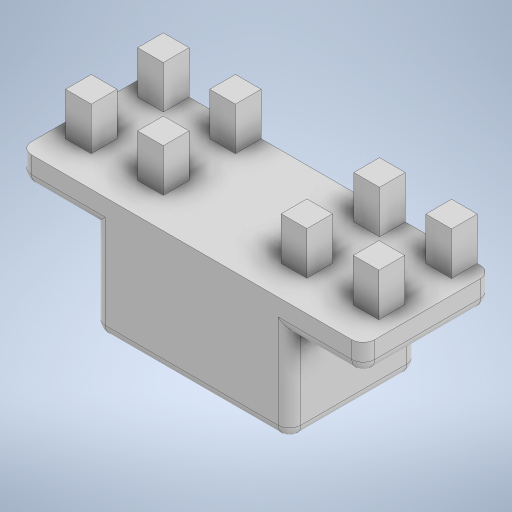
# Autodesk Inventor part: Platform
Saved by Autodesk Inventor 2024.1 (Build 281209000, 209)
## iProperties
Created: 2024-04-30
Part Number: Platform
Material: Generic
Document SubType Name: Modeling
Designer: cyan924
Density: 1 g/cm^3
Appearance: Default
Author: cyan924
Autodesk Inventor part; units mm, degrees
ref_plane "YZ Plane" through (0, 0, 0) normal (1, 0, 0) x (0, 1, 0)
ref_plane "XZ Plane" through (0, 0, 0) normal (0, 1, 0) x (-1, 0, 0)
ref_plane "XY Plane" through (0, 0, 0) normal (0, 0, 1) x (1, 0, 0)
sketch "Sketch1" plane through (0, 0, 0) normal (0, 1, 0) x (-1, 0, 0)
  line L0 (0, 0) -> (34.2, 0)
  line L1 (34.2, 0) -> (34.2, -22.5)
  line L2 (34.2, -22.5) -> (0, -22.5)
  line L3 (0, -22.5) -> (0, 0)
  line L4 (5, -17.5) -> (29.2, -17.5)
  line L5 (29.2, -17.5) -> (29.2, -5)
  line L6 (29.2, -5) -> (5, -5)
  line L7 (5, -5) -> (5, -17.5)
  dimension "d64" = 24.2
  dimension "d65" = 12.5
  dimension "d66" = 5
  dimension "d67" = 5
  dimension "d68" = 5
  dimension "d69" = 5
  constraints: 16 end point, 4 parallel, 2 horizontal, 2 perpendicular
  measures "d64" distance between parallel lines of L5 L7
  measures "d65" distance of L4.end L5.end
  measures "d66" distance between parallel lines of L1 L5
  measures "d67" distance between parallel lines of L3 L7
  measures "d68" distance between parallel lines of L0 L6
  measures "d69" distance between parallel lines of L2 L4
extrude "Extrusion4" add sketch "Sketch1" along normal blind 16.4
sketch "Sketch6" plane through (0, 16.4, 0) normal (0, 1, 0) x (1, 0, 0)
  line L0 (0, 0) -> (0, 22.5) projected
  line L1 (-34.2, 0) -> (0, 0) projected
  line L2 (-47.1, 22.5) -> (12.9, 22.5)
  line L3 (12.9, 22.5) -> (12.9, 0)
  line L4 (12.9, 0) -> (-47.1, 0)
  line L5 (-47.1, 0) -> (-47.1, 22.5)
  line L6 (0, 22.5) -> (-34.2, 22.5) projected
  point P0 (-17.1, 0)
  point P1 (15.9799, 21.8)
  point P2 (-17.1, 22.5)
  point P3 (-17.1, 22.5)
  dimension "d75" = 60
  dimension "d77" = 0
  constraints: 8 end point, 2 midpoint, 2 parallel, 1 horizontal, 1 perpendicular, 2 other
  measures "d75" distance between parallel lines of L3 L5
  measures "d77" distance of point (-17.1, 22.5) point (-17.1, 22.5)
extrude "Extrusion6" add sketch "Sketch6" along normal blind 5
sketch "Sketch7" plane through (0, 21.4, 0) normal (0, 1, 0) x (1, 0, 0)
  line L0 (-47.1, 22.5) -> (-47.1, 0) projected
  line L1 (-6.75, 22.5) -> (-6.75, 18)
  line L2 (-2.25, 22.5) -> (-2.25, 18)
  line L3 (-2.25, 18) -> (-6.75, 18)
  line L4 (-6.75, 22.5) -> (-2.25, 22.5)
  line L5 (12.9, 22.5) -> (-47.1, 22.5) projected
  line L6 (-31.95, 22.5) -> (-31.95, 18)
  line L7 (-27.45, 22.5) -> (-27.45, 18)
  line L8 (-27.45, 18) -> (-31.95, 18)
  line L9 (-31.95, 22.5) -> (-27.45, 22.5)
  line L10 (-40.05, 22.5) -> (-40.05, 18)
  line L11 (-40.05, 18) -> (-44.55, 18)
  line L12 (-44.55, 22.5) -> (-44.55, 18)
  line L13 (-44.55, 22.5) -> (-40.05, 22.5)
  line L14 (10.35, 22.5) -> (10.35, 18)
  line L15 (5.85, 22.5) -> (5.85, 18)
  line L16 (10.35, 18) -> (5.85, 18)
  line L17 (5.85, 22.5) -> (10.35, 22.5)
  line L18 (-6.85, 9.9) -> (-6.85, 5.4)
  line L19 (-2.35, 9.9) -> (-2.35, 5.4)
  line L20 (-2.35, 5.4) -> (-6.85, 5.4)
  line L21 (-6.85, 9.9) -> (-2.35, 9.9)
  line L22 (-27.45, 9.9) -> (-27.45, 5.4)
  line L23 (-31.95, 9.9) -> (-27.45, 9.9)
  line L24 (-27.45, 5.4) -> (-31.95, 5.4)
  line L25 (-31.95, 9.9) -> (-31.95, 5.4)
  line L26 (-40.05, 9.9) -> (-40.05, 5.4)
  line L27 (-44.55, 9.9) -> (-44.55, 5.4)
  line L28 (-40.05, 5.4) -> (-44.55, 5.4)
  line L29 (-44.55, 9.9) -> (-40.05, 9.9)
  line L30 (10.25, 9.9) -> (10.25, 5.4)
  line L31 (5.75, 9.9) -> (10.25, 9.9)
  line L32 (5.75, 9.9) -> (5.75, 5.4)
  line L33 (10.25, 5.4) -> (5.75, 5.4)
  point P0 (0, 0)
  point P1 (-2.25, 20.25)
  point P2 (-6.75, 20.25)
  point P3 (-4.5, 18)
  point P4 (-4.5, 22.5)
  point P5 (-31.95, 20.25)
  point P6 (-27.45, 20.25)
  point P7 (-29.7, 18)
  point P8 (-29.7, 22.5)
  point P9 (-44.55, 20.25)
  point P10 (-42.3, 18)
  point P11 (-40.05, 20.25)
  point P12 (10.35, 20.25)
  point P13 (5.85, 20.25)
  point P14 (8.1, 18)
  point P15 (-6.85, 7.65)
  point P16 (-2.35, 7.65)
  point P17 (-4.6, 5.4)
  point P18 (-4.6, 9.9)
  point P19 (-31.95, 7.65)
  point P20 (-29.7, 9.9)
  point P21 (-29.7, 5.4)
  point P22 (-27.45, 7.65)
  point P23 (-40.05, 7.65)
  point P24 (-44.55, 7.65)
  point P25 (-42.3, 5.4)
  point P26 (10.25, 7.65)
  point P27 (8, 5.4)
  point P28 (5.75, 7.65)
  point P29 (-27.45, 22.5)
  point P30 (-31.95, 22.5)
  dimension "d123" = 4.5
  dimension "d124" = 4.5
  dimension "d128" = 0
  dimension "d130" = 4.5
  dimension "d131" = 4.5
  dimension "d137" = 0
  dimension "d138" = 4.5
  dimension "d139" = 4.5
  dimension "d141" = 8.1
  dimension "d142" = 4.5
  dimension "d143" = 4.5
  dimension "d145" = 0
  dimension "d146" = 8.1
  dimension "d147" = 0
  dimension "d150" = 4.5
  dimension "d151" = 4.5
  dimension "d153" = 4.5
  dimension "d154" = 4.5
  dimension "d156" = 4.5
  dimension "d157" = 4.5
  dimension "d158" = 8.1
  dimension "d159" = 4.5
  dimension "d160" = 4.5
  dimension "d161" = 8.1
  dimension "d168" = 0
  dimension "d169" = 8.1
  dimension "d170" = 8.1
  dimension "d172" = 8.1
  dimension "d173" = 8.1
  constraints: 64 end point, 28 midpoint, 8 perpendicular, 8 vertical, 4 horizontal
  measures "d123" distance of L1.start L1.end
  measures "d124" distance between parallel lines of L2 L1
  measures "d128" distance between parallel lines of L5 L4
  measures "d130" distance of L9.start L8.end
  measures "d131" distance between parallel lines of L7 L6
  measures "d137" distance between parallel lines of L5 L9
  measures "d138" distance of L12.start L12.end
  measures "d139" distance between parallel lines of L10 L12
  measures "d141" distance between parallel lines of L6 L10
  measures "d142" distance of L17.start L15.end
  measures "d143" distance between parallel lines of L14 L15
  measures "d145" distance between parallel lines of L5 L13
  measures "d146" distance between parallel lines of L2 L15
  measures "d147" distance between parallel lines of L5 L17
  measures "d150" distance of L21.start L20.end
  measures "d151" distance between parallel lines of L19 L18
  measures "d153" distance of L23.start L25.end
  measures "d154" distance between parallel lines of L22 L25
  measures "d156" distance of L29.start L28.end
  measures "d157" distance between parallel lines of L26 L27
  measures "d158" distance between parallel lines of L25 L26
  measures "d159" distance of L32.start L32.end
  measures "d160" distance between parallel lines of L30 L32
  measures "d161" distance between parallel lines of L19 L32
  measures "d168" distance between parallel lines of L12 L27
  measures "d169" distance from line of point (-42.3, 18) L29
  measures "d170" distance of point (-29.7, 18) point (-29.7, 9.9)
  measures "d172" distance between parallel lines of L3 L21
  measures "d173" distance between parallel lines of L16 L31
extrude "Extrusion7" add sketch "Sketch7" along normal blind 7.5
sketch "Sketch8" plane through (-34.2, 0, -22.5) normal (-1, 0, 0) x (0, 0, 1)
  line L0 (17.5, 0) -> (17.5, 16.4) projected
  line L1 (5, 16.4) -> (17.5, 16.4) projected
  line L2 (17.5, 6.4) -> (5, 6.4)
  line L3 (5, 6.4) -> (5, 16.4)
  line L4 (5, 16.4) -> (17.5, 16.4)
  line L5 (17.5, 16.4) -> (17.5, 6.4)
  point P0 (22.5, 0)
  dimension "d176" = 10
  constraints: 8 end point, 2 parallel, 1 horizontal, 1 perpendicular, 1 point on line
  measures "d176" distance between parallel lines of L1 L2
extrude "Extrusion8" cut sketch "Sketch8" against normal blind 7.5
fillet "Fillet2" radius 2 21 edges at (-17.1, 0, -22.5) (-34.2, 0, -11.25) (0, 0, -11.25) (-17.1, 0, 0) (0, 8.2, -22.5) (6.45, 16.4, -22.5) (12.9, 16.4, -11.25) (6.45, 16.4, 0) (0, 8.2, 0) (-34.2, 8.2, -22.5) (-40.65, 16.4, -22.5) (-47.1, 16.4, -11.25) (-40.65, 16.4, 0) (-34.2, 8.2, 0) (12.9, 18.9, -22.5) (12.9, 18.9, 0) (-47.1, 18.9, -22.5) (-47.1, 18.9, 0) (-34.2, 11.4, -5) (-34.2, 6.4, -11.25) (-34.2, 11.4, -17.5)
equation "\"d141\" = gap"
equation "\"box\" = 4.5"
equation "\"walllength\" = 1"
equation "\"gap\" = 8.1"
equation "\"d34\" = 4.6"
equation "\"d35\" = 8"
equation "\"offset\" = 5"
equation "\"d44\" = 4.6"
equation "\"d89\" = 4.6"
equation "\"d126\" = 4.6"
equation "\"d134\" = 4.6"
equation "\"d135\" = 8"
equation "\"d140\" = 4.6"
equation "\"d144\" = 4.6"
equation "\"d162\" = 4.6"
equation "\"d163\" = 4.6"
equation "\"d164\" = 8"
equation "\"d165\" = 4.6"
equation "\"d166\" = 4.6"
equation "\"d167\" = 4.6"
body "Solid2"
